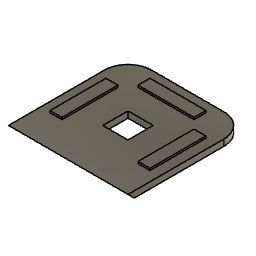
biosensorTop v2 (Autodesk Fusion 360 design; units mm, degrees)
Autodesk Fusion 360 part; units mm, degrees
sketch "Sketch1" plane through (0, 0, 0) normal (0, 0, 1) x (1, 0, 0)
  line L0 (0, 0) -> (38, 0)
  line L1 (38, 0) -> (38, 38)
  line L2 (38, 38) -> (0, 38)
  line L3 (0, 38) -> (0, 0)
  dimension "d1" = 38
  dimension "d2" = 38
  constraint horizontal L0
  constraint vertical L1
  constraint horizontal L2
  constraint vertical L3
  constraint coincident L0.start L3.end
  measures "d1" distance of L0.start L0.end
  measures "d2" distance of L0.start L2.end
extrude "Extrude1" add sketch "Sketch1" along normal blind 2
sketch "Sketch2" plane through (0, 0, 2) normal (0, 0, 1) x (-1, 0, 0)
  line L0 (0, -38) -> (0, 0)
  line L1 (0, 0) -> (-38, 0)
  line L2 (-38, 0) -> (-38, -38)
  line L3 (-38, -38) -> (0, -38)
  line L4 (-23, -23) -> (-23, -15)
  line L5 (-23, -15) -> (-15, -15)
  line L6 (-15, -15) -> (-15, -23)
  line L7 (-15, -23) -> (-23, -23)
  dimension "d6" = 8
  dimension "d7" = 8
  dimension "d8" = 8
  dimension "d9" = 15
  dimension "d10" = 15
  constraint perpendicular L4 L5
  constraint perpendicular L5 L6
  measures "d6" distance of L4.start L4.end
  measures "d7" distance of L4.end L5.end
  measures "d8" distance of L5.end L6.end
  measures "d9" distance of L3 L7
  measures "d10" distance of L0 L6
extrude "Extrude2" cut sketch "Sketch2" against normal blind 7 contours L4 L5 L6 L7
sketch "Sketch3" plane through (0, 0, 2) normal (0, 0, 1) x (-1, 0, 0)
  line L0 (-23, -15) -> (-15, -15)
  line L1 (-15, -15) -> (-15, -23)
  line L2 (-15, -23) -> (-23, -23)
  line L3 (-23, -23) -> (-23, -15)
  line L4 (0, -38) -> (0, 0)
  line L5 (0, 0) -> (-38, 0)
  line L6 (-38, 0) -> (-38, -38)
  line L7 (-38, -38) -> (0, -38)
  line L8 (-15, -23) -> (-15, -28)
  line L9 (-15, -28) -> (-10, -28)
  line L10 (-10, -28) -> (-28, -28)
  line L11 (-28, -28) -> (-28, -10)
  line L12 (-28, -10) -> (-10, -10)
  line L13 (-10, -10) -> (-10, -28)
  line L14 (-31, -28) -> (-35, -28)
  line L15 (-35, -28) -> (-35, -10)
  line L16 (-35, -10) -> (-31, -10)
  line L17 (-31, -10) -> (-31, -28)
  line L18 (-19, -28) -> (-19, -10)
  line L19 (-28, -28) -> (-10, -10)
  line L20 (-28, -31) -> (-28, -35)
  line L21 (-10, -31) -> (-28, -31)
  line L22 (-28, -35) -> (-10, -35)
  line L23 (-10, -35) -> (-10, -31)
  line L24 (-7, -10) -> (-7, -28)
  line L25 (-7, -28) -> (-3, -28)
  line L26 (-3, -28) -> (-3, -10)
  line L27 (-3, -10) -> (-7, -10)
  line L28 (-31.1, -27.9) -> (-34.9, -27.9)
  line L29 (-34.9, -27.9) -> (-34.9, -10.1)
  line L30 (-34.9, -10.1) -> (-31.1, -10.1)
  line L31 (-31.1, -10.1) -> (-31.1, -27.9)
  line L32 (-27.9, -31.1) -> (-27.9, -34.9)
  line L33 (-10.1, -31.1) -> (-27.9, -31.1)
  line L34 (-27.9, -34.9) -> (-10.1, -34.9)
  line L35 (-10.1, -34.9) -> (-10.1, -31.1)
  line L36 (-6.9, -27.9) -> (-3.1, -27.9)
  line L37 (-6.9, -10.1) -> (-6.9, -27.9)
  line L38 (-3.1, -27.9) -> (-3.1, -10.1)
  line L39 (-3.1, -10.1) -> (-6.9, -10.1)
  dimension "d13" = 5
  dimension "d14" = 5
  dimension "d15" = 18
  dimension "d16" = 18
  dimension "d17" = 4
  dimension "d18" = 3
  dimension "d19" = 0.1
  dimension "d20" = 0.1
  dimension "d21" = 0.1
  dimension "d22" = 0.1
  constraint coincident L1.end L2.start
  constraint perpendicular L2 L8
  constraint perpendicular L8 L9
  constraint horizontal L10
  constraint vertical L11
  constraint horizontal L12
  constraint vertical L13
  constraint horizontal L14
  constraint vertical L15
  constraint horizontal L16
  constraint vertical L17
  constraint midpoint L10 L18.start
  constraint midpoint L12 L18.end
  constraint symmetric L14.start L19 L20.start
  constraint symmetric L14.end L19 L20.end
  constraint symmetric L15.end L19 L22.end
  constraint symmetric L16.end L19 L21.start
  constraint symmetric L14.start L18 L24.end
  constraint symmetric L14.end L18 L25.end
  constraint symmetric L15.end L18 L26.end
  constraint symmetric L16.end L18 L24.start
  constraint horizontal L28
  constraint vertical L29
  constraint horizontal L30
  constraint vertical L31
  constraint symmetric L19 L28.start L32.start
  constraint symmetric L19 L28.end L32.end
  constraint symmetric L19 L29.end L34.end
  constraint symmetric L19 L30.end L33.start
  constraint symmetric L18 L28.start L36.start
  constraint symmetric L18 L28.end L36.end
  constraint symmetric L18 L29.end L38.end
  constraint symmetric L18 L30.end L37.start
  measures "d13" distance of L1.end L8.end
  measures "d14" distance of L8.end L9.end
  measures "d15" distance of L9.end L10.end
  measures "d16" distance of L9.end L12.end
  measures "d17" distance of L14.start L14.end
  measures "d18" distance of L11 L17
  measures "d19" distance of L15 L29
  measures "d20" distance of L16 L30
  measures "d21" distance of L17 L31
  measures "d22" distance of L14 L28
extrude "Extrude3" add sketch "Sketch3" along normal blind 0.6 contours L28 L29 L30 L31 | L32 L33 L34 L35 | L36 L37 L38 L39
fillet "Fillet1" radius 7.5 2 edges at (0, 38, 1) (38, 38, 1)
chamfer "Chamfer2" distance 2 angle 45 1 edges at (19, 0, 0)
